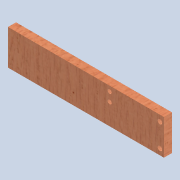
# Autodesk Inventor part: 0005-10-008
Saved by Autodesk Inventor 2020 (Build 240168000, 168)
## iProperties
Created: 2020-12-18
Part Number: 0005-10-008
Material: Wood (Maple)
Document SubType Name: Modeling
Designer: Iulian Bors
Density: 0.67 g/cm^3
Appearance: White Oak - Natural Medium Gloss
Mass: 28.7728 g
Surface Area: 142.034 cm^2
Volume: 42.9445 cm^3
Author: Iulian Bors
Subject: 008
Autodesk Inventor part; units mm, degrees
ref_plane "YZ Plane" through (0, 0, 0) normal (1, 0, 0) x (0, 1, 0)
ref_plane "XZ Plane" through (0, 0, 0) normal (0, 1, 0) x (-1, 0, 0)
ref_plane "XY Plane" through (0, 0, 0) normal (0, 0, 1) x (1, 0, 0)
sketch "Sketch1" plane through (0, 0, 0) normal (0, 0, 1) x (1, 0, 0)
  line L0 (-77.5, 17.5) -> (77.5, 17.5)
  line L1 (77.5, 17.5) -> (77.5, -17.5)
  line L2 (77.5, -17.5) -> (-77.5, -17.5)
  line L3 (-77.5, -17.5) -> (-77.5, 17.5)
  point P0 (0, 0)
  point P1 (0, 17.5)
  point P2 (-77.5, 0)
  dimension "d0" = 155
  dimension "d1" = 35
  constraints: 8 end point, 2 midpoint, 2 parallel, 1 horizontal, 1 horizontal alignment, 1 perpendicular, 1 vertical alignment
  measures "d0" distance of L0.start L0.end
  measures "d1" distance of L2.end L0.start
extrude "Extrusion1" add sketch "Sketch1" along normal blind 8
sketch "Sketch4" plane through (0, 0, 8) normal (0, 0, 1) x (1, 0, 0)
  line L0 (-73.5, -11.5) -> (73.5, -11.5) construction
  line L1 (73.5, -11.5) -> (73.5, 11.5) construction
  line L2 (73.5, 11.5) -> (-73.5, 11.5) construction
  line L3 (-73.5, 11.5) -> (-73.5, -11.5) construction
  line L4 (-77.5, 17.5) -> (-77.5, -17.5) construction
  line L5 (77.5, 17.5) -> (-77.5, 17.5) construction
  point P0 (0, 0)
  point P1 (-73.5, 0)
  point P2 (-77.5, 0)
  point P3 (0, 11.5)
  point P4 (0, 17.5)
  dimension "d19" = 4
  dimension "d20" = 6
  constraints: 8 end point, 4 midpoint, 2 parallel, 1 horizontal, 1 horizontal alignment, 1 perpendicular, 1 vertical alignment
  measures "d19" distance from line of L4 point (-73.5, 0)
  measures "d20" distance between parallel lines of L5 L2
hole "Hole1" at (73.5, -11.5, 8) at (73.5, 11.5, 8) direction (0, 0, -1) diameter 4.5 end through all
sketch "Sketch5" plane through (0, 0, 8) normal (0, 0, 1) x (1, 0, 0)
  circle A0 centre (23.5, 3.5) radius 1.75 projected
  circle A1 centre (23.5, 12.5) radius 1.75 projected
  point P0 (0, 0)
hole "Hole2" at (23.5, 3.5, 8) at (23.5, 12.5, 8) direction (0, 0, -1) diameter 4 end through all
body "Solid1"
